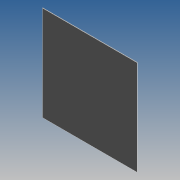
# Autodesk Inventor part: P002_plancher
Saved by Autodesk Inventor 2020 (Build 240168000, 168)
## iProperties
Created: 2021-09-24
Part Number: P002_plancher
Material: Générique
Document SubType Name: Modeling
Designer: gabri
Density: 1 g/cm^3
Appearance: Par défaut
Author: gabri
Autodesk Inventor part; units mm, degrees
ref_plane "YZ Plane" through (0, 0, 0) normal (1, 0, 0) x (0, 1, 0)
ref_plane "XZ Plane" through (0, 0, 0) normal (0, 1, 0) x (-1, 0, 0)
ref_plane "XY Plane" through (0, 0, 0) normal (0, 0, 1) x (1, 0, 0)
sketch "Esquisse2" plane through (0, 0, 0) normal (0, 1, 0) x (-1, 0, 0)
  line L0 (4000, 4000) -> (-4000, 4000)
  line L1 (-4000, 4000) -> (-4000, -4000)
  line L2 (-4000, -4000) -> (4000, -4000)
  line L3 (4000, -4000) -> (4000, 4000)
  line L4 (0, -5600) -> (0, 5600) construction
  line L5 (-5600, 0) -> (5600, 0) construction
  point P0 (0, 0)
  dimension "d0" = 8000
  dimension "d1" = 8000
  dimension "d2" = 4000
  dimension "d3" = 4000
  constraints: 8 end point, 2 parallel, 1 horizontal, 1 perpendicular
  measures "d0" distance of L0.end L1.end
  measures "d1" distance of L1.end L2.end
  measures "d2" distance between parallel lines of L4 L3
  measures "d3" distance between parallel lines of L5 L2
extrude "Extrusion1" add sketch "Esquisse2" along normal blind 40
